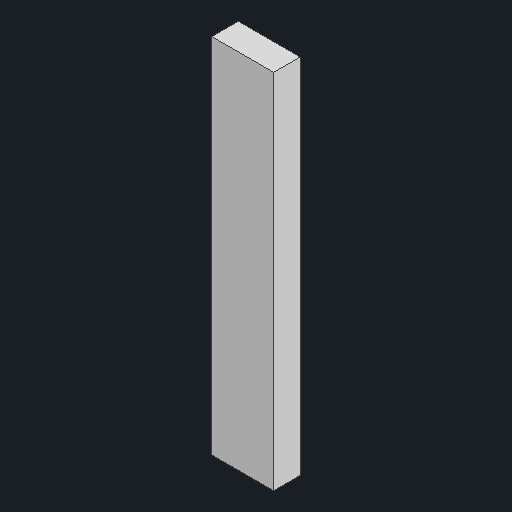
# Autodesk Inventor part: 2x4x20.5
Saved by Autodesk Inventor 2026 (Build 300175000, 175)
## iProperties
Created: 2024-09-20
Part Number: 2x4x20.5
Material: Generic
Document SubType Name: Modeling
Designer: User
Density: 1 g/cm^3
Appearance: Default
Author: User
Autodesk Inventor part; units mm, degrees
ref_plane "YZ Plane" through (0, 0, 0) normal (1, 0, 0) x (0, 1, 0)
ref_plane "XZ Plane" through (0, 0, 0) normal (0, 1, 0) x (-1, 0, 0)
ref_plane "XY Plane" through (0, 0, 0) normal (0, 0, 1) x (1, 0, 0)
sketch "Sketch1" plane through (0, 0, 0) normal (0, 0, 1) x (1, 0, 0)
  line L0 (0, 215.9) -> (590.55, 215.9) projected
  line L1 (0, 177.0325) -> (0, 215.9) projected
  line L2 (-590.55, -304.8) -> (628.65, -304.8) projected
  line L3 (0, 215.9) -> (0, -304.8)
  line L4 (88.9, -304.8) -> (88.9, 215.9)
  point P0 (0, 0)
  dimension "d0" = 88.9
  constraints: 4 end point, 3 point on line, 2 perpendicular
  measures "d0" distance between parallel lines of L3 L4
extrude "Extrusion1" add sketch "Sketch1" against normal blind 38.1
body "Solid1"
